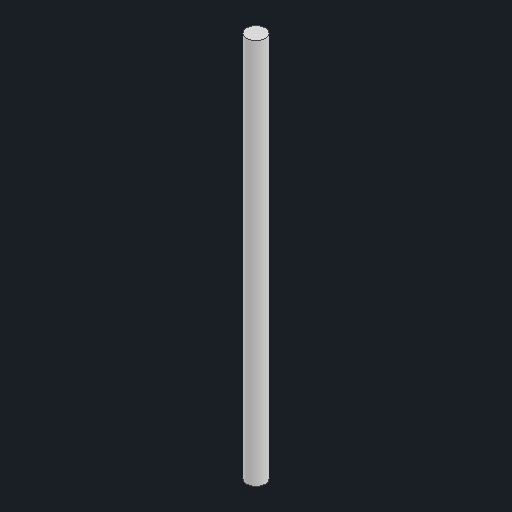
# Autodesk Inventor part: ReserviorPistonRod
Saved by Autodesk Inventor 2024 (Build 280153000, 153)
## iProperties
Created: 2025-02-08
Part Number: ReserviorPistonRod
Material: Generic
Document SubType Name: Modeling
Designer: Tommy Rohmann
Density: 1 g/cm^3
Appearance: Default
Author: Tommy Rohmann
Autodesk Inventor part; units mm, degrees
ref_plane "YZ Plane" through (0, 0, 0) normal (1, 0, 0) x (0, 1, 0)
ref_plane "XZ Plane" through (0, 0, 0) normal (0, 1, 0) x (-1, 0, 0)
ref_plane "XY Plane" through (0, 0, 0) normal (0, 0, 1) x (1, 0, 0)
sketch "ReserviorPistonRod" plane through (0, 0, 0) normal (0, 0, 1) x (1, 0, 0)
  line L0 (99.4709, 260.9643) -> (99.4709, 523.6257)
  line L1 (99.4709, 523.6257) -> (86.7709, 523.6257)
  line L2 (86.7709, 523.6257) -> (86.7709, 260.9643)
  line L3 (86.7709, 260.9643) -> (99.4709, 260.9643)
  line L4 (93.1209, 523.6257) -> (93.1209, 260.9643)
  line L5 (86.7709, 291.6983) -> (99.4709, 291.6983)
  line L6 (99.4709, 498.2257) -> (86.7709, 498.2257)
  point P0 (25.0598, 339.6513)
  dimension "d191" = 12.7
  dimension "d202" = 30.734
  dimension "d544" = 206.5274
  dimension "d545" = 25.4
  measures "d191" distance between parallel lines of L0 L2
  measures "d202" distance between parallel lines of L3 L5
  measures "d544" distance between parallel lines of L5 L6
  measures "d545" distance between parallel lines of L1 L6
derived "LAYOUT.ipt"
sketch "Sketch1" plane through (0, 0, 0) normal (0, 0, 1) x (1, 0, 0)
  line L0 (99.4709, 260.9643) -> (99.4709, 523.6257)
  line L1 (99.4709, 523.6257) -> (86.7709, 523.6257)
  line L2 (86.7709, 523.6257) -> (86.7709, 260.9643)
  line L3 (86.7709, 260.9643) -> (99.4709, 260.9643)
  line L4 (93.1209, 523.6257) -> (93.1209, 260.9643)
  line L5 (86.7709, 291.6983) -> (99.4709, 291.6983)
  line L6 (99.4709, 498.2257) -> (86.7709, 498.2257)
revolve "Revolution1" add sketch "Sketch1" angle 360 about axis through (93.1209, 523.6257, 0) along (0, -1, 0) contours L3 L2 L5 L4 | L5 L2 L6 L4 | L6 L2 L1 L4
body "Solid1"
